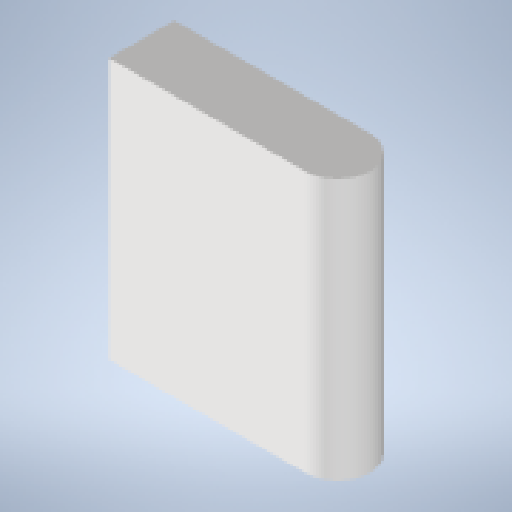
# Autodesk Inventor part: FixedClamp
Saved by Autodesk Inventor 2023 (Build 270158000, 158)
## iProperties
Created: 2023-09-03
Part Number: FixedClamp
Material: Generic
Document SubType Name: Modeling
Designer: Felix
Density: 1 g/cm^3
Appearance: Default
Author: Felix
Autodesk Inventor part; units mm, degrees
ref_plane "YZ Plane" through (0, 0, 0) normal (1, 0, 0) x (0, 1, 0)
ref_plane "XZ Plane" through (0, 0, 0) normal (0, 1, 0) x (-1, 0, 0)
ref_plane "XY Plane" through (0, 0, 0) normal (0, 0, 1) x (1, 0, 0)
sketch "Sketch1" plane through (0, 0, 0) normal (0, 1, 0) x (-1, 0, 0)
  arc A0 (0, 2.5) -> (0, -2.5) centre (0, 0) ccw
  line L0 (0, -2.5) -> (15, -2.5)
  line L1 (15, -2.5) -> (15, 2.5)
  line L2 (15, 2.5) -> (0, 2.5)
  dimension "d0" = 5
  dimension "d1" = 15
  constraints: 6 end point, 2 point on circle, 2 tangent, 1 centre point, 1 coincident, 1 horizontal, 1 parallel, 1 perpendicular
  measures "d0" diameter of A0
  measures "d1" distance from line of L1 A0.centre
extrude "Extrusion1" add sketch "Sketch1" along normal blind 25
sketch "Sketch2" plane through (-15, 0, 2.5) normal (0, 0, 1) x (1, 0, 0)
  line L0 (0, 0) -> (15, 0) construction
  line L1 (15, 0) -> (15, 25) construction
  line L2 (0, 25) -> (15, 25) construction
  line L3 (0, 0) -> (0, 25) construction
  line L4 (0, 0) -> (0, 25) construction
  line L5 (15, 6.5) -> (0, 6.5) construction
  line L6 (0, 6.5) -> (0, 18.5) construction
  line L7 (0, 18.5) -> (15, 18.5) construction
  line L8 (15, 18.5) -> (15, 6.5) construction
  line L9 (15, 12.5) -> (0, 12.5) construction
  line L10 (15, 6.5) -> (0, 0) construction
  line L11 (15, 0) -> (0, 0) construction
  line L12 (0, 6.5) -> (15, 0) construction
  line L13 (15, 25) -> (0, 25) construction
  line L14 (15, 25) -> (0, 18.5) construction
  line L15 (0, 25) -> (15, 18.5) construction
  line L16 (11.5, 21.75) -> (3.5, 21.75) construction
  line L17 (11.5, 23.35) -> (3.5, 23.35)
  line L18 (3.5, 20.15) -> (11.5, 20.15)
  arc A0 (11.5, 20.15) -> (11.5, 23.35) centre (11.5, 21.75) ccw
  arc A1 (3.5, 23.35) -> (3.5, 20.15) centre (3.5, 21.75) ccw
  line L19 (11.5, 3.25) -> (3.5, 3.25) construction
  line L20 (11.5, 1.65) -> (3.5, 1.65)
  line L21 (3.5, 4.85) -> (11.5, 4.85)
  arc A2 (11.5, 1.65) -> (11.5, 4.85) centre (11.5, 3.25) ccw
  arc A3 (3.5, 4.85) -> (3.5, 1.65) centre (3.5, 3.25) ccw
  point P0 (7.5, 21.75)
  point P1 (7.5, 21.75)
  point P2 (7.5, 3.25)
  point P3 (7.5, 3.25)
  dimension "d4" = 12
  dimension "d5" = 3.2
  dimension "d6" = 8
  constraints: 34 end point, 8 point on circle, 8 symmetric about line, 4 centre point, 4 midpoint, 4 tangent, 3 parallel, 2 coincident, 2 horizontal, 2 point on line, 1 perpendicular, 3 other
  measures "d4" distance between parallel lines of L5 L7
  measures "d5" diameter of A1
  measures "d6" distance of L16.start L16.end
extrude "Extrusion2" cut sketch "Sketch2" against normal through all
ref_plane "Work Plane2" through (-15, 12.5, 2.5) normal (0, 1, 0) x (1, 0, 0)
body "Solid1"
